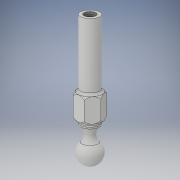
# Autodesk Inventor part: Component 41(Push Rod Base)
Saved by Autodesk Inventor 2018 (Build 220112000, 112)
## iProperties
Created: 2023-04-01
Part Number: Component 41(Push Rod Base)
Material: Generic
Document SubType Name: Modeling
Designer: Habib Mohamed
Density: 1 g/cm^3
Appearance: Default
Author: Habib Mohamed
Autodesk Inventor part; units mm, degrees
ref_plane "YZ Plane" through (0, 0, 0) normal (1, 0, 0) x (0, 1, 0)
ref_plane "XZ Plane" through (0, 0, 0) normal (0, 1, 0) x (-1, 0, 0)
sketch "Sketch1" plane through (0, 0, 0) normal (1, 0, 0) x (0, 1, 0)
  arc A0 (-2.5, 0) -> (1.8333, -1.6997) centre (0, 0) ccw
  line L0 (5.254, -2) -> (25, -2)
  line L1 (25, -2) -> (25, -1.25)
  arc A1 (4.8632, -1.8119) -> (1.8333, -1.6997) centre (3.3, -3.0594) ccw
  arc A2 (4.8632, -1.8119) -> (5.254, -2) centre (5.254, -1.5) ccw
  line L2 (25, -1.25) -> (5, -1.25)
  line L3 (5, -1.25) -> (5, 0)
  line L4 (5, 0) -> (-2.5, 0)
  point P0 (4.9964, -2)
  dimension "d0" = 5
  dimension "d2" = 3.3
  dimension "d3" = 4
  dimension "d4" = 25
  dimension "d6" = 0.5
  dimension "d8" = 20
  dimension "d9" = 0.75
  dimension "d10" = 19.746
  dimension "d11" = 5
  constraints: 10 end point, 7 point on circle, 3 centre point, 3 tangent, 2 coincident, 2 parallel, 2 point on line, 1 horizontal, 1 perpendicular
  measures "d0" diameter of A0
  measures "d2" horizontal distance of point (0, 0) point (3.3, -3.059)
  measures "d3" diameter of A1
  measures "d4" distance from line of L1 point (0, 0)
  measures "d6" radius of A2
  measures "d8" distance of L1.end L2.end
  measures "d9" distance of L0.end L1.end
  measures "d10" distance of L0.start L0.end
  measures "d11" distance from line of point (0, 0) L3
revolve "Revolution1" add sketch "Sketch1" angle 360 about axis through (0, 5, 0) along (0, -1, 0)
thread "Thread1" size "M2.5x0.35" class "6H" standard "ANSI Metric M Profile" full length
ref_plane "Work Plane1" through (0, 11, 0) normal (0, 1, 0) x (1, 0, 0)
sketch "Sketch2" plane through (0, 11, 0) normal (0, 1, 0) x (1, 0, 0)
  line L0 (1.4434, 2.5) -> (2.8868, 0)
  line L1 (2.8868, 0) -> (1.4434, -2.5)
  line L2 (1.4434, -2.5) -> (-1.4434, -2.5)
  line L3 (-1.4434, -2.5) -> (-2.8868, 0)
  line L4 (-2.8868, 0) -> (-1.4434, 2.5)
  line L5 (-1.4434, 2.5) -> (1.4434, 2.5)
  circle A0 centre (0, 0) radius 1.25 projected
  point P0 (0, 0)
  point P1 (0, 0)
  dimension "d16" = 5
  constraints: 12 end point, 1 coincident, 13 other
  measures "d16" distance between parallel lines of L2 L5
extrude "Extrusion1" add sketch "Sketch2" against normal blind 5
sketch "Sketch3" plane through (0, 11, 0) normal (0, 1, 0) x (1, 0, 0)
  circle A0 centre (0, 0) radius 2.5
  line L0 (-2.8868, 0) -> (-1.4434, 2.5) projected
  constraints: 1 centre point, 1 coincident, 1 tangent
extrude "Extrusion2" cut sketch "Sketch3" against normal blind 40 draft 35 and the other way blind 40 keep common part
sketch "Sketch4" plane through (0, 6, 0) normal (0, -1, 0) x (1, 0, 0)
  arc A0 (2.1651, 1.25) -> (0, 2.5) centre (0, 0) ccw projected
  circle A1 centre (0, 0) radius 2.5 projected
  point P0 (0, 0)
extrude "Extrusion3" cut sketch "Sketch4" against normal blind 40 draft 35 and the other way blind 40 keep common part
fillet "Fillet1" radius 0.5 2 edges at (0, 11, 2) (0, 6, 2)
body "Solid1"
